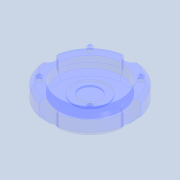
# Autodesk Inventor part: cpd_1.9_p0_v12
Saved by Autodesk Inventor 2021 (Build 250183000, 183)
## iProperties
Created: 2022-10-19
Part Number: cpd_1.9_p0_v12
Material: Generic
Document SubType Name: Modeling
Designer: to172
Density: 1 g/cm^3
Appearance: Clear - Blue
Author: to172
Autodesk Inventor part; units mm, degrees
ref_plane "YZ Plane" through (0, 0, 0) normal (1, 0, 0) x (0, 1, 0)
ref_plane "XZ Plane" through (0, 0, 0) normal (0, 1, 0) x (-1, 0, 0)
ref_plane "XY Plane" through (0, 0, 0) normal (0, 0, 1) x (1, 0, 0)
sketch "Sketch1" plane through (0, 0, 0) normal (0, 0, 1) x (1, 0, 0)
  line L0 (0, 0) -> (0, 12.75) construction
  line L1 (0, 0) -> (13.9342, 0) construction
  line L2 (0, 0) -> (0, -3)
  line L3 (0, -3) -> (12.5, -3)
  line L4 (12.5, -3) -> (12.5, 3.25)
  line L5 (12.5, 3.25) -> (9.075, 3.25)
  line L6 (9.075, 3.25) -> (9.075, 0)
  line L7 (9.075, 0) -> (0, 0)
  line L8 (3, 0) -> (5, 0)
  line L9 (5, 0) -> (5, -0.5)
  line L10 (5, -0.5) -> (3, -0.5)
  line L11 (3, -0.5) -> (3, 0)
  dimension "d0" = 3
  dimension "d1" = 5
  dimension "d2" = 0.5
  dimension "d3" = 9.075
  dimension "d4" = 12.5
  dimension "d5" = 3.25
  dimension "d6" = 3
  constraints: 24 end point, 5 perpendicular, 2 horizontal, 2 parallel, 2 point on line, 2 vertical, 1 collinear
  measures "d0" distance between parallel lines of L11 L0
  measures "d1" distance between parallel lines of L0 L9
  measures "d2" distance between parallel lines of L1 L10
  measures "d3" distance between parallel lines of L0 L6
  measures "d4" distance between parallel lines of L0 L4
  measures "d5" distance between parallel lines of L5 L1
  measures "d6" distance between parallel lines of L1 L3
revolve "Revolution1" add sketch "Sketch1" angle 360 about axis through (0, 0, 0) along (0, 1, 0) contours L7 L11 L10 L9 L6 L5 L4 L3 L2
chamfer "Chamfer1" distance 2 angle 45 1 edges at (-12.5, -3, 0)
chamfer "Chamfer2" distance 1 angle 45 1 edges at (-12.5, 3.25, 0)
sketch "Sketch2" plane through (0, 3.25, 0) normal (0, 1, 0) x (1, 0, 0)
  circle A0 centre (0, 0) radius 12.5 projected
  circle A1 centre (0, 0) radius 12.5 projected
  circle A2 centre (0, -12.5) radius 2.5
  line L0 (0, 0) -> (0, -12.5) construction
  point P0 (2.4875, -12.25)
  point P1 (-2.4875, -12.25)
  dimension "d14" = 5
  constraints: 2 end point, 1 centre point, 1 vertical, 1 vertical alignment, 1 other
  measures "d14" diameter of A2
extrude "Extrusion1" cut sketch "Sketch2" against normal through all contours A2 A0 picked at (0, -11.6481)
pattern_circular "Circular Pattern1" count 4 over 360 about axis through (0, -10, 0) along (0, 1, 0) of "Extrusion1"
sketch "Sketch3" plane through (0, 3.25, 12.5) normal (0, 1, 0) x (1, 0, 0)
  line L0 (0, 12.5) -> (0, -7.7808) construction
  line L1 (0, 12.5) -> (13.1543, -0.6543) construction
  circle A0 centre (7.4246, 5.0754) radius 0.75
  dimension "d20" = 45
  dimension "d21" = 1.5
  dimension "d22" = 10.5
  constraints: 4 end point, 1 centre point, 1 point on line, 1 vertical
  measures "d20" angle of L1 L0
  measures "d21" diameter of A0
  measures "d22" distance of L0.start A0.centre
extrude "Extrusion2" add sketch "Sketch3" along normal blind 1.5
chamfer "Chamfer3" distance 0.35 angle 45 1 edges at (6.6746, 4.75, 7.4246)
pattern_circular "Circular Pattern2" count 4 over 360 about axis through (0, -10, 0) along (0, 1, 0) of "Extrusion2", "Chamfer3"
body "Solid1"
